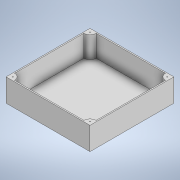
# Autodesk Inventor part: caja_cuboLed
Saved by Autodesk Inventor 2021 (Build 250183000, 183)
## iProperties
Created: 2022-06-13
Part Number: caja_cuboLed
Material: Genérico
Document SubType Name: Modeling
Designer: Dell
Density: 1 g/cm^3
Appearance: Valor por defecto
Author: Dell
Autodesk Inventor part; units mm, degrees
ref_plane "YZ Plane" through (0, 0, 0) normal (1, 0, 0) x (0, 1, 0)
ref_plane "XZ Plane" through (0, 0, 0) normal (0, 1, 0) x (-1, 0, 0)
ref_plane "XY Plane" through (0, 0, 0) normal (0, 0, 1) x (1, 0, 0)
sketch "Boceto1" plane through (0, 0, 0) normal (0, 1, 0) x (-1, 0, 0)
  line L0 (-103, 103) -> (103, 103)
  line L1 (103, 103) -> (103, -103)
  line L2 (103, -103) -> (-103, -103)
  line L3 (-103, -103) -> (-103, 103)
  line L4 (-103, 103) -> (103, -103) construction
  line L5 (103, 103) -> (-103, -103) construction
  point P0 (0, 0)
  dimension "d0" = 206
  dimension "d1" = 206
  constraints: 12 end point, 2 midpoint, 2 parallel, 1 horizontal, 1 perpendicular
  measures "d0" distance of L1.end L2.end
  measures "d1" distance of L0.end L1.end
extrude "Extrusión1" add sketch "Boceto1" along normal blind 56
shell "Vaciado1" thickness 3 removed faces 1 at (34.3333, 56, 34.3333)
sketch "Boceto2" plane through (-100, 3, -100) normal (0, 1, 0) x (1, 0, 0)
  line L0 (200, 0) -> (0, 0) projected
  arc A0 (0, -15) -> (15, 0) centre (0, 0) ccw
  line L1 (200, -200) -> (200, 0) projected
  arc A1 (185, 0) -> (200, -15) centre (200, 0) ccw
  line L2 (200, -200) -> (0, -200) projected
  arc A2 (200, -185) -> (185, -200) centre (200, -200) ccw
  line L3 (0, -200) -> (0, 0) projected
  arc A3 (15, -200) -> (0, -185) centre (0, -200) ccw
  line L4 (0, 0) -> (15, 0)
  line L5 (0, 0) -> (0, -15)
  line L6 (200, 0) -> (200, -15)
  line L7 (200, 0) -> (185, 0)
  line L8 (200, -200) -> (200, -185)
  line L9 (200, -200) -> (185, -200)
  line L10 (0, -200) -> (0, -185)
  line L11 (0, -200) -> (15, -200)
  point P0 (100, -100)
  dimension "d5" = 30
  dimension "d6" = 30
  dimension "d7" = 30
  dimension "d8" = 30
  constraints: 16 end point, 8 point on circle, 7 point on line, 4 centre point, 3 coincident
  measures "d5" diameter of A0
  measures "d6" diameter of A1
  measures "d7" diameter of A2
  measures "d8" diameter of A3
extrude "Extrusión2" add sketch "Boceto2" along normal blind 53 contours L1 A1 L0 | A0 L3 L0 | L1 L2 A2 | A3 L2 L3
sketch "Boceto3" plane through (0, 56, 0) normal (0, 1, 0) x (1, 0, 0)
  line L0 (85, 100) -> (103, 100)
  line L1 (103, -103) -> (103, 103) projected
  line L2 (100, -85) -> (100, 85) projected
  line L3 (100, 85) -> (100, 100)
  line L4 (100, 100) -> (116.202, 100) construction
  arc A0 (85, 100) -> (100, 85) centre (100, 100) ccw projected
  line L5 (89.3934, 89.3934) -> (89.3934, 100)
  line L6 (89.3934, 89.3934) -> (100, 89.3934)
  line L7 (89.3934, 100) -> (100, 89.3934)
  line L8 (89.3934, 89.3934) -> (100, 100)
  circle A1 centre (94.6967, 94.6967) radius 1
  circle A2 centre (-94.6967, 94.6967) radius 1
  circle A3 centre (-94.6967, -94.6967) radius 1
  circle A4 centre (94.6967, -94.6967) radius 1
  point P0 (0, 0)
  dimension "d12" = 2
  dimension "d15" = 360
  constraints: 14 end point, 4 centre point, 4 perpendicular, 4 point on line, 2 horizontal, 1 midpoint, 1 point on circle, 9 other
  measures "d12" diameter of A1
hole "Agujero1" at (-94.6967, 56, -94.6967) at (-94.6967, 56, 94.6967) at (94.6967, 56, 94.6967) at (94.6967, 56, -94.6967) direction (0, -1, 0) diameter 2 depth 25 tip angle 118
